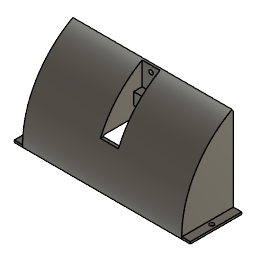
redirigir aire (Autodesk Fusion 360 design; units mm, degrees)
Autodesk Fusion 360 part; units mm, degrees
sketch "Boceto2" plane through (0, 0, 0) normal (1, 0, 0) x (0, 1, 0)
  line L0 (68.4642, 1.8454) -> (35.7202, 62)
  arc A0 (35.7202, 62) -> (0, 0) centre (68.4642, 1.8454) ccw
  line L1 (0, 0) -> (2.0007, 0)
  arc A1 (36.6764, 60.2434) -> (2.0007, 0) centre (68.4642, 1.8454) ccw
  line L2 (0, 0) -> (-30, 0)
  line L3 (-30, 0) -> (-30, 76.7154)
  line L4 (-30, 76.7154) -> (35, 76.7154)
  line L5 (35, 76.7154) -> (35.7202, 62)
  dimension "d22" = 2
  dimension "d23" = 66.489
  dimension "d24" = 62
  constraint coincident L1.start A0
  constraint coincident A0.end L1.start
  constraint horizontal L1
  constraint coincident L0.start A0.centre
  constraint coincident L0 A1.start
  constraint concentric A0 A1
  constraint horizontal L2
  constraint perpendicular L2 L3
  constraint perpendicular L3 L4
  measures "d22" distance of A0 A1
  measures "d23" radius of A1
  measures "d24" distance of L0.end L1
extrude "Extruir1" add sketch "Boceto2" along normal mid plane 109 contours L0 A0 L1 A1
sketch "Boceto3" plane through (54.5, 0, 0) normal (1, 0, 0) x (0, 1, 0)
  line L0 (36.6764, 60.2434) -> (35.7202, 62)
  arc A0 (35.7202, 62) -> (0, 0) centre (68.4642, 1.8454) ccw
  line L1 (36.6764, 60.2434) -> (36.6764, 0)
  line L2 (36.6764, 0) -> (0, 0)
  line L3 (0, 0) -> (2.0007, 0)
  arc A1 (36.6764, 60.2434) -> (2.0007, 0) centre (68.4642, 1.8454) ccw
  constraint coincident L0.start L1.start
  constraint vertical L1
  constraint coincident A0.end L2.end
  constraint perpendicular L1 L2
extrude "Extruir2" add sketch "Boceto3" along normal blind 2
mirror "Simetría1" about plane through (0, 0, 0) normal (1, 0, 0) of "Extruir2"
sketch "Boceto6" plane through (0, 0, 45) normal (0, 0, 1) x (1, 0, 0)
  circle A0 centre (0, 31.68) radius 1.4142
  line L0 (-6.35, 34.68) -> (6.35, 34.68)
  line L1 (6.35, 34.68) -> (6.35, 28.68)
  line L2 (6.35, 28.68) -> (-6.35, 28.68)
  line L3 (-6.35, 28.68) -> (-6.35, 34.68)
  line L4 (-6.35, 34.68) -> (6.35, 28.68) construction
  line L5 (6.35, 34.68) -> (-6.35, 28.68) construction
  line L6 (-7.85, 28.68) -> (-7.85, 34.68)
  line L7 (-6.35, 28.68) -> (-6.35, 6.0685)
  line L8 (-6.35, 6.0685) -> (-7.85, 6.0685)
  line L9 (-7.85, 6.0685) -> (-7.85, 28.68)
  line L10 (-7.85, 36.6684) -> (-7.85, 34.68)
  line L11 (6.35, 6.0685) -> (7.6183, 6.0685)
  line L12 (6.35, 28.68) -> (6.35, 6.0685)
  line L13 (7.6183, 36.6684) -> (-7.85, 36.6684)
  line L14 (7.6183, 36.6684) -> (7.6183, 6.0685)
  line L15 (-6.35, 6.0685) -> (6.35, 6.0685)
  point P0 (0, 31.68)
  dimension "d13" = 1.5
  dimension "d62" = 2.8284
  dimension "d63" = 34.68
  dimension "d64" = 6.35
  dimension "d65" = 6.35
  dimension "d66" = 3
  dimension "d67" = 15.4683
  dimension "d68" = 30.5999
  dimension "d69" = 28.6115
  constraint horizontal L0
  constraint perpendicular L0 L1
  constraint parallel L0 L2
  constraint parallel L1 L3
  constraint coincident L4 P0
  constraint coincident L5 P0
  constraint perpendicular L7 L8
  constraint perpendicular L11 L14
  constraint perpendicular L7 L15
  constraint perpendicular L8 L9
  constraint perpendicular L10 L13
  constraint perpendicular L13 L14
  constraint perpendicular L11 L12
  constraint parallel L6 L12
  constraint parallel L7 L14
  constraint collinear L1 L12
  constraint coincident P0 A0.centre
  constraint coincident L1.end L2.start
  constraint equal L1 L6
  constraint equal L7 L9
  measures "d13" distance of L2.end L6.start
  measures "d62" diameter of A0
  measures "d63" distance of origin L0
  measures "d64" distance of origin L1
  measures "d65" distance of P0 L1
  measures "d66" distance of P0 L0
  measures "d67" distance of L10 L14
  measures "d68" distance of L11 L13.start
  measures "d69" distance of L0 L11
extrude "Extruir4" add sketch "Boceto6" against normal blind 16 contours L0 L1 L3 L6 L7 L8 L9 L10 L11 L12 L13 L14 | L0 L1 L2 L3
sketch "Boceto7" plane through (0, 0, 45) normal (0, 0, 1) x (-1, 0, 0)
sketch "Boceto8" plane through (0, 0, 0) normal (0, 0, -1) x (1, 0, 0)
  line L0 (56.5, 0) -> (-56.5, 0)
  line L1 (56.5, -0.0439) -> (62.5, -0.0439)
  line L2 (62.5, -0.0439) -> (62.5, -36.6764)
  line L3 (62.5, -36.6764) -> (56.5, -36.6764)
  line L4 (56.5, -36.6764) -> (56.5, -0.0439)
  line L5 (59.5, -36.6764) -> (59.5, -0.0439)
  circle A0 centre (59.5, -18.3601) radius 1.5
  line L6 (-54.5, -2.0007) -> (54.5, -2.0007)
  line L7 (54.5, -2.0007) -> (54.5, -36.6764)
  line L8 (54.5, -36.6764) -> (56.5, -36.6764)
  line L9 (56.5, -36.6764) -> (56.5, 0)
  line L10 (-56.5, 0) -> (-56.5, -36.6764)
  line L11 (-56.5, -36.6764) -> (-54.5, -36.6764)
  line L12 (-54.5, -36.6764) -> (-54.5, -2.0007)
  dimension "d31" = 6
  dimension "d33" = 3
  constraint horizontal L1
  constraint vertical L2
  constraint horizontal L3
  constraint vertical L4
  constraint midpoint L3 L5.start
  constraint midpoint L1 L5.end
  constraint coincident L5 A0.centre
  constraint midpoint L5 A0.centre
  constraint coincident L3.end L4.start
  measures "d31" distance of L1.start L1.end
  measures "d33" diameter of A0
extrude "Extruir7" add sketch "Boceto8" against normal blind 1.5 contours L1 L3 L4 L5 A0 L9 | L1 L2 L3 L5 A0
ref_plane "PlanoDeObra1" through (0, 0, 45) normal (0, 0, 1) x (1, 0, 0)
sketch "Boceto10" plane through (0, 0, 45) normal (0, 0, 1) x (1, 0, 0)
extrude "Extruir8" cut sketch "Boceto6" along normal blind 27 contours A0 | L0 L1 L3 L6 L7 L8 L9 L10 L11 L12 L13 L14 | L0 L1 L2 L3 | L2 L7 L12 L15
extrude "Extruir9" cut sketch "Boceto6" against normal blind 17 contours L2 L7 L12 L15
sketch "Boceto11" plane through (0, 0, 29) normal (0, 0, -1) x (1, 0, 0)
  line L0 (7.6183, -7.773) -> (6.35, -7.773)
  line L1 (6.35, -7.773) -> (6.35, -28.68)
  line L2 (6.35, -28.68) -> (-6.35, -28.68)
  line L3 (-6.35, -28.68) -> (-6.35, -7.773)
  line L4 (-6.35, -7.773) -> (-7.85, -7.773)
  line L5 (-7.85, -7.773) -> (-7.85, -36.6684)
  line L6 (-7.85, -36.6684) -> (7.6183, -36.6684)
  line L7 (7.6183, -36.6684) -> (7.6183, -7.773)
  circle A0 centre (0, -31.68) radius 1.4142
  line L8 (-6.35, -28.68) -> (6.2342, -28.68)
  line L9 (6.2342, -28.68) -> (6.2342, -36.6684)
  line L10 (6.2342, -36.6684) -> (-6.35, -36.6684)
  line L11 (-6.35, -36.6684) -> (-6.35, -28.68)
  constraint horizontal L8
  constraint vertical L9
  constraint horizontal L10
  constraint vertical L11
  constraint coincident L6 L9.end
  constraint coincident L2.end L3.start
extrude "Extruir10" cut sketch "Boceto11" against normal blind 7.5 contours L2 L6 L8 L9 L10 L11
extrude "Extruir11" add sketch "Boceto6" along normal blind 17 contours L0 L1 L3 L6 L7 L8 L9 L10 L11 L12 L13 L14
sketch "Boceto12" plane through (56.5, 0, 0) normal (1, 0, 0) x (0, 1, 0)
  line L0 (0.0439, 0) -> (0.0439, 1.5)
  line L1 (0.0439, 1.5) -> (36.6764, 1.5)
  line L2 (36.6764, 1.5) -> (36.6764, 60.2434)
  line L3 (36.6764, 60.2434) -> (35.7202, 62)
  arc A0 (35.7202, 62) -> (0, 0) centre (68.4642, 1.8454) ccw
  line L4 (0, 0) -> (0.0439, 0)
extrude "Extruir12" cut sketch "Boceto2" along normal mid plane 140 contours A0 L2 L3 L4 L5
sketch "Boceto13" plane through (0, 34.68, 0) normal (0, -1, 0) x (1, 0, 0)
  line L0 (-6.35, 61.422) -> (-6.35, 45)
  line L1 (-6.35, 45) -> (6.35, 45)
  line L2 (6.35, 45) -> (6.35, 61.422)
  line L3 (6.35, 61.422) -> (-6.35, 61.422)
  circle A0 centre (0, 57) radius 1.5
  dimension "d57" = 3
  measures "d57" diameter of A0
extrude "Extruir15" cut 1 faces at (-7.85, 36.3523, 61.4194) along direction (1, 0, 0) blind 18
extrude "Extruir16" cut sketch "Boceto13" against normal blind 7 contours A0
extrude "Extruir17" cut 1 faces at (-2.1167, 6.0685, 29.3907) along direction (0, -1, 0) blind 10
mirror "Simetría5" about plane through (0, 0, 0) normal (1, 0, 0) of "Extruir7"
